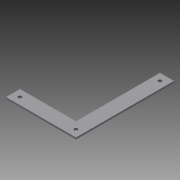
# Autodesk Inventor part: topLayer
Saved by Autodesk Inventor 2014 (Build 180170000, 170)
## iProperties
Created: 2014-10-04
Part Number: topLayer
Material: Generic
Document SubType Name: Modeling
Designer: Rachel
Density: 1 g/cm^3
Appearance: Default
Author: Rachel
Autodesk Inventor part; units mm, degrees
ref_plane "YZ Plane" through (0, 0, 0) normal (1, 0, 0) x (0, 1, 0)
ref_plane "XZ Plane" through (0, 0, 0) normal (0, 1, 0) x (-1, 0, 0)
ref_plane "XY Plane" through (0, 0, 0) normal (0, 0, 1) x (1, 0, 0)
sketch "Sketch1" plane through (0, 0, 0) normal (0, 1, 0) x (-1, 0, 0)
  line L0 (-63.5, -88.9) -> (63.5, -88.9)
  line L1 (63.5, -88.9) -> (63.5, 88.9)
  line L2 (63.5, 88.9) -> (-63.5, 88.9)
  line L3 (-63.5, 88.9) -> (-63.5, -88.9)
  line L4 (-63.5, -88.9) -> (63.5, 88.9) construction
  line L5 (63.5, -88.9) -> (-63.5, 88.9) construction
  line L6 (63.5, -88.9) -> (-38.1, -88.9)
  line L7 (-38.1, -88.9) -> (-38.1, 63.5)
  line L8 (-38.1, 63.5) -> (63.5, 63.5)
  line L9 (63.5, 63.5) -> (63.5, -88.9)
  point P0 (0, 0)
  dimension "d0" = 127
  dimension "d1" = 177.8
  dimension "d2" = 101.6
  dimension "d3" = 152.4
  constraints: 20 end point, 4 parallel, 2 horizontal, 2 midpoint, 2 perpendicular
  measures "d0" distance of L2.end L1.end
  measures "d1" distance of L2.end L0.start
  measures "d2" distance of L7.end L8.end
  measures "d3" distance of L6.end L7.end
extrude "Extrusion1" add sketch "Sketch1" along normal blind 3.175 contours L3 L2 L1 L8 L7 L0
sketch "Sketch2" plane through (0, 3.175, 0) normal (0, 1, 0) x (1, 0, 0)
  line L0 (-63.5, -63.5) -> (-63.5, -88.9) projected
  line L1 (-63.5, -88.9) -> (63.5, -88.9) projected
  line L2 (63.5, -88.9) -> (63.5, 88.9) projected
  line L3 (63.5, 88.9) -> (38.1, 88.9) projected
  line L4 (-63.5, -76.2) -> (63.5, -76.2) construction
  line L5 (50.8, 88.9) -> (50.8, -88.9) construction
  point P0 (0, 0)
  point P1 (-50.8, -76.2)
  point P2 (50.8, 76.2)
  point P3 (50.8, -76.2)
  dimension "d6" = 12.7
  dimension "d7" = 12.7
  constraints: 6 point on line, 4 end point, 2 midpoint, 2 perpendicular
  measures "d6" distance of L5.start point (50.8, 76.2)
  measures "d7" distance from line of L0 point (-50.8, -76.2)
hole "Hole1" at (-50.8, 3.175, 76.2) at (50.8, 3.175, -76.2) at (50.8, 3.175, 76.2) direction (0, -1, 0) diameter 6.477 end through all
body "Solid1"
